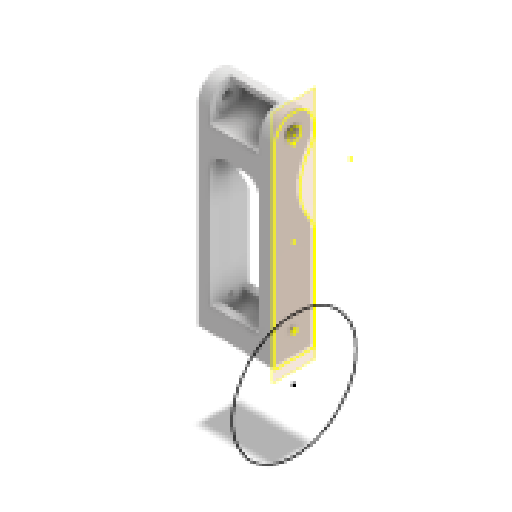
# Autodesk Inventor part: swingarmV3
Saved by Autodesk Inventor 2025 (Build 290162000, 162)
## iProperties
Created: 2024-10-22
Part Number: swingarmV3
Material: Generic
Document SubType Name: Modeling
Designer: derm
Density: 1 g/cm^3
Appearance: Default
Author: derm
Autodesk Inventor part; units mm, degrees
ref_plane "Work Plane3" through (13.5242, 0, 0) normal (1, 0, 0) x (0, 0, -1)
sketch "Sketch1" plane through (0, 0, 0) normal (1, 0, 0) x (0, 1, 0)
  circle A0 centre (0, 0) radius 4.25
  line L0 (0, 0) -> (-109.1267, 0) construction
  line L1 (0, 12.461) -> (-109.1267, 12.461)
  line L2 (-109.1267, -12.461) -> (0, -12.461)
  arc A1 (0, -12.461) -> (0, 12.461) centre (0, 0) ccw
  arc A2 (-109.1267, 12.461) -> (-109.1267, -12.461) centre (-109.1267, 0) ccw
  circle A3 centre (-109.1267, 0) radius 1.5
  line L3 (-121.5877, 0) -> (-185.4539, 0) construction
  line L4 (-121.5877, -6.7248) -> (-185.4539, -6.7248)
  line L5 (-185.4539, 6.7248) -> (-121.5877, 6.7248)
  arc A4 (-121.5877, -6.7248) -> (-121.5877, 6.7248) centre (-121.5877, 0) ccw
  arc A5 (-185.4539, 6.7248) -> (-185.4539, -6.7248) centre (-185.4539, 0) ccw
  point P0 (-54.5633, 0)
  point P1 (-153.5208, 0)
  point P2 (-119.7731, -6.4754)
  point P3 (-119.7731, 6.4754)
  dimension "d0" = 8.5
  dimension "d8" = 3
  constraints: 16 end point, 9 point on circle, 8 tangent, 6 centre point, 2 coincident, 2 horizontal, 2 midpoint, 2 parallel
  measures "d0" diameter of A0
  measures "d8" diameter of A3
extrude "Extrusion1" add sketch "Sketch1" against normal blind 8 contours A1 L2 A2 A4 L1 | A4 A2
sketch "Sketch2" plane through (0, 0, 0) normal (1, 0, 0) x (0, 0, -1)
  arc A0 (-12.461, -109.1267) -> (12.461, -109.1267) centre (0, -109.1267) ccw projected
  line L0 (12.461, -109.1267) -> (12.461, 0) projected
  arc A1 (12.461, 0) -> (-12.461, 0) centre (0, 0) ccw projected
  line L1 (-12.461, 0) -> (-12.461, -109.1267) projected
  circle A2 centre (0, 0) radius 4.25 projected
  circle A3 centre (0, 0) radius 9.1207
  constraints: 1 centre point, 1 coincident
extrude "Extrusion2" cut sketch "Sketch2" against normal blind 2 contours A3
sketch "Sketch3" plane through (-2, 0, 0) normal (1, 0, 0) x (0, 0, -1)
  circle A0 centre (0, 0) radius 9.1207 projected
  circle A1 centre (0, 0) radius 4.25 projected
  circle A2 centre (0, 0) radius 3.25
  dimension "d5" = 6.5
  constraints: 1 centre point, 1 coincident
  measures "d5" diameter of A2
extrude "Extrusion3" add sketch "Sketch3" against normal blind 3 contours A1
ref_plane "Work Plane1" through (15.5, 0, 0) normal (1, 0, 0) x (0, 0, -1)
mirror "Mirror1" about plane through (15.5, 0, 0) normal (1, 0, 0)
sketch "Sketch4" plane through (-8, 0, 0) normal (-1, 0, 0) x (0, 0, 1)
  arc A0 (-12.461, -109.1267) -> (12.461, -109.1267) centre (0, -109.1267) ccw projected
  line L0 (12.461, -109.1267) -> (12.461, 0) projected
  arc A1 (12.461, 0) -> (-12.461, 0) centre (0, 0) ccw projected
  line L1 (-12.461, 0) -> (-12.461, -109.1267) projected
  circle A2 centre (0, -109.1267) radius 1.5 projected
  circle A3 centre (0, 0) radius 4.25 projected
  line L2 (12.461, -109.1267) -> (12.461, -124.3041)
  line L3 (12.461, -124.3041) -> (-12.461, -124.3041)
  line L4 (-12.461, -124.3041) -> (-12.461, -109.1267)
  arc A4 (-7.419, -109.1267) -> (7.419, -109.1267) centre (0, -109.1267) ccw
  line L5 (-12.461, -109.1267) -> (-7.419, -109.1267)
  line L6 (-1.5, -109.1267) -> (1.5, -109.1267)
  line L7 (7.419, -109.1267) -> (12.461, -109.1267)
  circle A5 centre (0, -164.1149) radius 36.8515
  line L8 (0, -109.1267) -> (0, -164.1149) construction
  point P0 (-12.461, -123.7794)
  point P1 (12.461, -123.7794)
  constraints: 14 end point, 4 parallel, 4 point on circle, 3 horizontal, 3 perpendicular, 2 centre point, 2 coincident, 1 vertical
extrude "Extrusion4" add sketch "Sketch4" against normal up to surface (47 mm away) contours L5 A4 L7 A0 | A0 L2 L3 L4
sketch "Sketch5" plane through (39, 0, 0) normal (1, 0, 0) x (0, 0, -1)
  line L0 (12.461, -124.3041) -> (12.461, 0) projected
  arc A0 (12.461, 0) -> (-12.461, 0) centre (0, 0) ccw projected
  line L1 (-12.461, -124.3041) -> (-12.461, 0) projected
  circle A1 centre (0, -109.1267) radius 1.5 projected
  circle A2 centre (0, 0) radius 4.25 projected
  arc A3 (12.461, -9.7623) -> (12.461, -54.6283) centre (36.2892, -32.1953) ccw
  line L2 (-12.461, -124.3041) -> (12.461, -124.3041) projected
  constraints: 2 point on circle, 2 point on line, 1 centre point, 2 other
extrude "Extrusion5" cut sketch "Sketch5" against normal through all contours A3 L0
fillet "Fillet1" radius 12.7 4 edges at (35, -9.7623, -12.461) (-4, -9.7623, -12.461) (35, -54.6283, -12.461) (-4, -54.6283, -12.461)
sketch "Sketch6" plane through (0, 0, 0) normal (1, 0, 0) x (0, 0, -1)
  arc A0 (12.461, -59.2) -> (9.9733, -51.6503) centre (-0.239, -59.2) ccw projected
  arc A1 (9.9733, -12.7404) -> (9.9733, -51.6503) centre (36.2892, -32.1953) ccw projected
  arc A2 (9.9733, -12.7404) -> (12.461, -5.1906) centre (-0.239, -5.1906) ccw projected
  line L0 (12.461, -5.1906) -> (12.461, 0) projected
  arc A3 (12.461, 0) -> (-12.461, 0) centre (0, 0) ccw projected
  line L1 (-12.461, 0) -> (-12.461, -109.1267) projected
  line L2 (-12.461, -109.1267) -> (-7.419, -109.1267) projected
  arc A4 (-7.419, -109.1267) -> (7.419, -109.1267) centre (0, -109.1267) ccw projected
  line L3 (7.419, -109.1267) -> (12.461, -109.1267) projected
  line L4 (12.461, -109.1267) -> (12.461, -59.2) projected
  circle A5 centre (0, -109.1267) radius 1.5 projected
  circle A6 centre (0, 0) radius 9.1207 projected
  arc A7 (12.461, 0) -> (-12.461, 0) centre (0, 0) ccw projected
  arc A8 (9.9733, -12.7404) -> (9.9733, -51.6503) centre (36.2892, -32.1953) ccw projected
  line L5 (3.5628, -32.1953) -> (-3.9488, -32.1953)
  line L6 (-3.9488, -32.1953) -> (-3.9488, -9.1207)
  circle A9 centre (0, 0) radius 9.1207 projected
  line L7 (0, 9.1207) -> (0, 12.461)
  line L8 (-3.9488, -24.1282) -> (4.5726, -24.1282)
  line L9 (0, -9.1207) -> (-12.461, -9.1207)
  line L10 (-3.9488, -32.1953) -> (-12.461, -32.1953)
  line L11 (-3.9488, -24.1282) -> (-12.461, -24.1282)
  point P0 (4.5726, -24.1282)
  constraints: 14 end point, 7 point on circle, 5 point on line, 3 horizontal, 3 perpendicular, 2 tangent, 1 parallel
extrude "Extrusion6" add sketch "Sketch6" along normal up to next contours L8 L6 L9 A6 L7 A3 L0 A2 A1 | L11 L1 L9 L6
fillet "Fillet2" [suppressed]
fillet "Fillet4" radius 10.16 4 edges at (0, -24.1282, -0.3119) (0, -24.1282, 8.2049) (31, -24.1282, -0.3119) (31, -24.1282, 8.2049)
ref_plane "Work Plane2" through (19.5242, 0, 0) normal (-1, 0, 0) x (0, 0, 1)
ref_plane "Work Plane5" through (41, 0, 0) normal (1, 0, 0) x (0, 0, -1)
sketch "Sketch16" plane through (41, 0, 0) normal (1, 0, 0) x (0, 0, -1)
  circle A0 centre (0, 0) radius 4.25 projected
  circle A1 centre (0, -109.1267) radius 1.5 projected
  line L0 (-12.461, -124.3041) -> (-12.461, 0) projected
  line L1 (-12.461, -124.3041) -> (12.461, -124.3041) projected
  line L2 (12.461, -124.3041) -> (12.461, -59.2) projected
  arc A2 (12.461, -59.2) -> (9.9733, -51.6503) centre (-0.239, -59.2) ccw projected
  arc A3 (9.9733, -12.7404) -> (9.9733, -51.6503) centre (36.2892, -32.1953) ccw projected
  arc A4 (9.9733, -12.7404) -> (12.461, -5.1906) centre (-0.239, -5.1906) ccw projected
  line L3 (12.461, -5.1906) -> (12.461, 0) projected
  arc A5 (12.461, 0) -> (-12.461, 0) centre (0, 0) ccw projected
  circle A6 centre (0, -139.0661) radius 39.579
  constraints: 1 centre point
sketch "Sketch7" plane through (19.5242, 0, 0) normal (-1, 0, 0) x (0, 0, 1)
  arc A0 (-9.9733, -51.6503) -> (-12.461, -59.2) centre (0.239, -59.2) ccw projected
  line L0 (-12.461, -59.2) -> (-12.461, -123.7794) projected
  arc A1 (12.461, -123.7794) -> (-12.461, -123.7794) centre (0, -164.1149) ccw projected
  line L1 (12.461, -123.7794) -> (12.461, 0) projected
  arc A2 (12.461, 0) -> (-12.461, 0) centre (0, 0) ccw projected
  line L2 (-12.461, 0) -> (-12.461, -5.1906) projected
  arc A3 (-9.9733, -51.6503) -> (-9.9733, -12.7404) centre (-36.2892, -32.1953) ccw projected
  circle A4 centre (0, 0) radius 4.25 projected
  circle A5 centre (0, -109.1267) radius 1.5 projected
  circle A6 centre (0, -164.1149) radius 4 projected
  circle A7 centre (0, -164.1149) radius 4.1
  arc A8 (-12.461, -164.1149) -> (12.461, -164.1149) centre (0, -164.1149) ccw
  line L3 (-12.461, -123.7794) -> (-12.461, -164.1149)
  line L4 (12.461, -164.1149) -> (12.461, -123.7794)
  arc A9 (-12.461, -5.1906) -> (-9.9733, -12.7404) centre (0.239, -5.1906) ccw projected
  dimension "d21" = 8.2
  constraints: 4 end point, 2 centre point, 2 coincident, 2 point on circle, 1 parallel, 1 tangent, 1 vertical
  measures "d21" diameter of A7
sketch "Sketch8" plane through (-8, 0, 0) normal (-1, 0, 0) x (0, 0, 1)
  circle A0 centre (0, -109.1267) radius 1.5 projected
  circle A1 centre (0, -109.1267) radius 3
  point P0 (0, 0)
  dimension "d25" = 6
  constraints: 1 centre point, 1 coincident
  measures "d25" diameter of A1
sketch "Sketch9" plane through (31, -109.1267, 12.461) normal (-1, 0, 0) x (0, 0, 1)
  arc A0 (-22.4343, 57.4764) -> (-16.0908, 74.8384) centre (-48.7503, 76.9313) ccw projected
  arc A1 (-22.4343, 57.4764) -> (-24.9221, 49.9266) centre (-12.2221, 49.9266) ccw projected
  line L0 (-24.9221, 0) -> (-24.9221, 49.9266) projected
  line L1 (-24.9221, 0) -> (-19.88, 0) projected
  arc A2 (-19.88, 0) -> (-5.042, 0) centre (-12.461, 0) ccw projected
  line L2 (-5.042, 0) -> (0, 0) projected
  line L3 (0, 109.1267) -> (0, 100.006) projected
  arc A3 (0, 109.1267) -> (-12.461, 121.5877) centre (-12.461, 109.1267) ccw projected
  circle A4 centre (-12.461, 0) radius 1.5 projected
  circle A5 centre (-12.461, 0) radius 1.5 projected
  arc A6 (-19.88, 0) -> (-5.042, 0) centre (-12.461, 0) ccw projected
  circle A7 centre (-12.461, 0) radius 7.419
  line L4 (-24.9221, 7.419) -> (0, 7.419)
  line L5 (0, 109.1267) -> (0, 0) projected
  line L6 (-16.0908, 74.8384) -> (0, 74.8384) projected
  line L7 (0, 74.8384) -> (0, 0) projected
  line L8 (-12.461, 100.006) -> (0, 100.006) projected
  line L9 (-12.461, 121.5877) -> (-12.461, 118.2473) projected
  arc A8 (-12.461, 100.006) -> (-12.461, 118.2473) centre (-12.461, 109.1267) ccw projected
  dimension "d46" = 12.92
  constraints: 1 centre point, 1 coincident
  measures "d46" distance from line of point (-5.595, 3.23) L3
sketch "Sketch12" plane through (78.3874, 0, 0) normal (1, 0, 0) x (0, 0, -1)
  line L0 (12.461, -123.7794) -> (12.461, -91.67) projected
  arc A0 (12.461, -91.67) -> (-12.461, -91.67) centre (0, -164.1149) ccw projected
  line L1 (-12.461, -91.67) -> (-12.461, -123.7794) projected
  arc A1 (12.461, -123.7794) -> (-12.461, -123.7794) centre (0, -164.1149) ccw projected
  circle A2 centre (0, -109.1267) radius 1.5 projected
  line L2 (12.461, -123.7794) -> (12.461, -164.1149) projected
  arc A3 (12.461, -123.7794) -> (-12.461, -123.7794) centre (0, -164.1149) ccw projected
  line L3 (-12.461, -164.1149) -> (-12.461, -123.7794) projected
  arc A4 (-12.461, -164.1149) -> (12.461, -164.1149) centre (0, -164.1149) ccw projected
  circle A5 centre (0, -164.1149) radius 4.1 projected
  point P0 (0, 0)
  point P1 (12.461, -123.7794)
  point P2 (-12.461, -123.7794)
sketch "Sketch13" plane through (90.3874, 0, 0) normal (1, 0, 0) x (0, 0, -1)
  circle A0 centre (0, -164.1149) radius 7 projected
  point P0 (0, 0)
sketch "Sketch14" plane through (31, -109.1267, -12.461) normal (0, 0, -1) x (-1, 0, 0)
  line L0 (-59.3874, -54.9882) -> (-59.3874, -26.1221) projected
  line L1 (-47.3874, -54.9882) -> (-59.3874, -54.9882) projected
  line L2 (-47.3874, -54.9882) -> (-47.3874, -14.6527) projected
  line L3 (11.4758, -14.6527) -> (-47.3874, -14.6527) projected
  line L4 (11.4758, -14.6527) -> (11.4758, -54.9882) projected
  line L5 (11.4758, -54.9882) -> (23.4873, -54.9882) projected
  line L6 (39, 49.9266) -> (39, 5.4577) projected
  line L7 (31, 49.9266) -> (39, 49.9266) projected
  line L8 (31, 0) -> (31, 49.9266) projected
  line L9 (31, 0) -> (0, 0) projected
  line L10 (0, 0) -> (0, 49.9266) projected
  line L11 (-19.2836, 49.9266) -> (0, 49.9266) projected
  line L12 (-8.9774, 40.6514) -> (-8.9774, -6.3546)
  line L13 (-8.9774, -6.3546) -> (-43.0529, -6.3546)
  arc A0 (-8.9774, 40.6514) -> (-43.0529, -6.3546) centre (62.2279, -46.8206) ccw
  point P0 (31, 109.1267)
  constraints: 4 end point, 2 point on circle, 1 centre point, 1 perpendicular, 1 vertical, 4 other
sketch "Sketch15" plane through (78.3874, 0, 0) normal (-1, 0, 0) x (0, 0, 1)
  arc A0 (12.461, -123.7794) -> (-12.461, -123.7794) centre (0, -164.1149) ccw projected
  line L0 (-12.461, -164.1149) -> (-12.461, -123.7794) projected
  arc A1 (-12.461, -164.1149) -> (12.461, -164.1149) centre (0, -164.1149) ccw projected
  line L1 (12.461, -123.7794) -> (12.461, -164.1149) projected
  circle A2 centre (0, -164.1149) radius 4.1 projected
  point P0 (0, 0)
body "Solid1"
